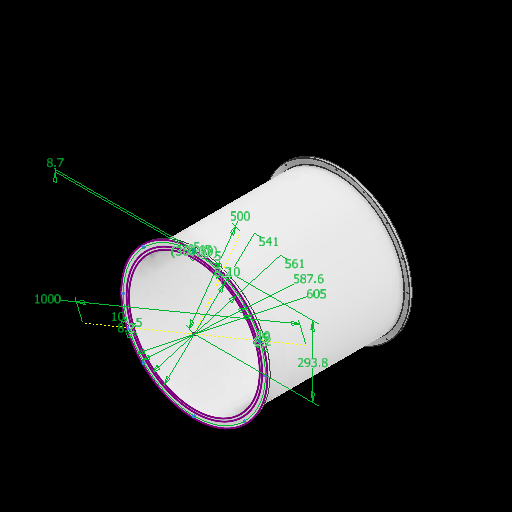
# Autodesk Inventor part: proteox_mx_approx
Saved by Autodesk Inventor 2026.1 (Build 301233000, 233)
## iProperties
Created: 2025-09-13
Part Number: proteox_mx_approx
Material: Stainless Steel
Document SubType Name: Modeling
Designer: drago
Density: 8 g/cm^3
Appearance: Smooth - White
Author: drago
Autodesk Inventor part; units mm, degrees
ref_plane "YZ Plane" through (0, 0, 0) normal (1, 0, 0) x (0, 1, 0)
ref_plane "XZ Plane" through (0, 0, 0) normal (0, 1, 0) x (-1, 0, 0)
ref_plane "XY Plane" through (0, 0, 0) normal (0, 0, 1) x (1, 0, 0)
sketch "Sketch6" plane through (0, 0, 0) normal (0, 0, 1) x (1, 0, 0)
  circle A0 centre (0, 0) radius 302.5
  circle A1 centre (0, 0) radius 280.5
  circle A2 centre (0, 0) radius 270.5
  circle A3 centre (0, 293.8) radius 5 construction
  circle A4 centre (0, 293.8) radius 2.5
  circle A5 centre (0, 293.8) radius 4.225 construction
  circle A6 centre (0, 0) radius 293.8 construction
  circle A7 centre (271.4358, 112.4324) radius 5 construction
  line L0 (0, 0) -> (191.3417, 461.9398) construction
  circle A8 centre (-271.4358, -112.4324) radius 5 construction
  circle A9 centre (112.4324, 271.4358) radius 5 construction
  line L1 (-267.0619, -110.6207) -> (-267.6799, -115.3144) construction
  line L2 (-267.6799, -115.3144) -> (-272.0538, -117.1262) construction
  line L3 (-272.0538, -117.1262) -> (-275.8097, -114.2441) construction
  line L4 (-275.8097, -114.2441) -> (-275.1918, -109.5504) construction
  line L5 (-275.1918, -109.5504) -> (-270.8179, -107.7386) construction
  line L6 (-270.8179, -107.7386) -> (-267.0619, -110.6207) construction
  line L7 (275.8097, 114.2441) -> (275.1918, 109.5504) construction
  line L8 (275.1918, 109.5504) -> (270.8179, 107.7386) construction
  line L9 (270.8179, 107.7386) -> (267.0619, 110.6207) construction
  line L10 (267.0619, 110.6207) -> (267.6799, 115.3144) construction
  line L11 (267.6799, 115.3144) -> (272.0538, 117.1262) construction
  line L12 (272.0538, 117.1262) -> (275.8097, 114.2441) construction
  line L13 (114.2441, 275.8097) -> (117.1262, 272.0538) construction
  line L14 (117.1262, 272.0538) -> (115.3144, 267.6799) construction
  line L15 (115.3144, 267.6799) -> (110.6207, 267.0619) construction
  line L16 (110.6207, 267.0619) -> (107.7386, 270.8179) construction
  line L17 (107.7386, 270.8179) -> (109.5504, 275.1918) construction
  line L18 (109.5504, 275.1918) -> (114.2441, 275.8097) construction
  circle A10 centre (112.4324, 271.4358) radius 2.5
  circle A11 centre (271.4358, 112.4324) radius 2.5
  circle A12 centre (-271.4358, -112.4324) radius 2.5
  circle A13 centre (-207.748, 207.748) radius 5 construction
  circle A14 centre (-207.748, 207.748) radius 4.225 construction
  circle A15 centre (-207.748, 207.748) radius 2.5
  circle A16 centre (-293.8, 0) radius 5 construction
  circle A17 centre (-293.8, 0) radius 4.225 construction
  circle A18 centre (-293.8, 0) radius 2.5
  circle A19 centre (-207.748, -207.748) radius 5 construction
  circle A20 centre (-207.748, -207.748) radius 4.225 construction
  circle A21 centre (-207.748, -207.748) radius 2.5
  circle A22 centre (0, -293.8) radius 5 construction
  circle A23 centre (0, -293.8) radius 4.225 construction
  circle A24 centre (0, -293.8) radius 2.5
  circle A25 centre (207.748, -207.748) radius 5 construction
  circle A26 centre (207.748, -207.748) radius 4.225 construction
  circle A27 centre (207.748, -207.748) radius 2.5
  circle A28 centre (293.8, 0) radius 5 construction
  circle A29 centre (293.8, 0) radius 4.225 construction
  circle A30 centre (293.8, 0) radius 2.5
  circle A31 centre (207.748, 207.748) radius 5 construction
  circle A32 centre (207.748, 207.748) radius 4.225 construction
  circle A33 centre (207.748, 207.748) radius 2.5
  line L19 (-461.9398, -191.3417) -> (461.9398, 191.3417) construction
  point P0 (0, 302.5)
  dimension "d31" = 605
  dimension "d34" = 561
  dimension "d35" = 541
  dimension "d36" = 10
  dimension "d37" = 8.7
  dimension "d38" = 293.8
  dimension "d39" = 5
  dimension "d40" = 8.45
  dimension "d47" = 587.6
  dimension "d48" = 10
  dimension "d49" = 500
  dimension "d53" = 10
  dimension "d54" = 10
  dimension "d55" = 8.2
  dimension "d56" = 8.2
  dimension "d57" = 8.2
  dimension "d58" = 5
  dimension "d59" = 5
  dimension "d60" = 5
  dimension "d63" = 360
  dimension "d77" = 1000
  constraints: 40 end point, 34 centre point, 26 coincident, 3 point on circle, 2 point on line, 1 midpoint, 88 other
  measures "d31" diameter of A0
  measures "d34" diameter of A1
  measures "d35" diameter of A2
  measures "d36" diameter of A3
  measures "d37" distance of point (0, 302.5) A3.centre
  measures "d38" distance of point (0, 0) A3.centre
  measures "d39" diameter of A4
  measures "d40" diameter of A5
  measures "d47" diameter of A6
  measures "d48" diameter of A7
  measures "d49" distance of L0.start L0.end
  measures "d53" diameter of A8
  measures "d54" diameter of A9
  measures "d55" distance between parallel lines of L2 L5
  measures "d56" distance between parallel lines of L8 L11
  measures "d57" distance between parallel lines of L14 L17
  measures "d58" diameter of A10
  measures "d59" diameter of A11
  measures "d60" diameter of A12
  measures "d77" distance of L19.start L19.end
extrude "Extrusion6" add sketch "Sketch6" against normal blind 600 contours A1 | A2
sketch "Sketch7" plane through (0, 0, -600) normal (0, 0, -1) x (-1, 0, 0)
  circle A0 centre (0, 0) radius 280.5 projected
  circle A1 centre (0, 0) radius 302.5
  dimension "d67" = 605
  constraints: 1 centre point, 1 coincident
  measures "d67" diameter of A1
extrude "Extrusion7" add sketch "Sketch7" against normal blind 12.2 contours A0 | A1
extrude "Extrusion8" cut sketch "Sketch6" against normal blind 600 contours A2
extrude "Extrusion9" add sketch "Sketch6" against normal blind 12.2 contours A0
extrude "Extrusion10" cut sketch "Sketch6" against normal blind 600 contours A4 | A10 | A11 | A12 | A15 | A18 | A21 | A24 | A27 | A30 | A33
fillet "Fillet2" radius 1 8 edges at (-302.5, 0, -12.2) (-302.5, 0, 0) (-280.5, 0, -12.2) (302.5, 0, -587.8) (302.5, 0, -600) (-280.5, 0, -587.8) (-270.5, 0, -600) (-270.5, 0, 0)
body "Solid2"
